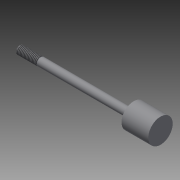
# Autodesk Inventor part: 021-DXP0000_rod
Saved by Autodesk Inventor 2014 SP2 (Build 180246200, 246)
## iProperties
Created: 2019-01-18
Part Number: 021-DXP0000_rod
Material: Generic
Catalog Web Link: www.cadenas.de
Description: Standard Air Cylinder_rod-Original Line - Standard Air Cylinders
Vendor: BIMBA
Document SubType Name: Modeling
Designer: psadmin
Manufacturer: BIMBA
Mass: 3.79157 g
Surface Area: 20.575 cm^2
Volume: 3.79157 cm^3
Density: 1 g/cm^3
Appearance: PSOLRGB-181-181-181
Category: PARTsolutions
Company: BIMBA
Title: 021-DXP0000_rod
Author: Cadenas PARTsolutions
Comments: Original Line - Standard Air Cylinders
PSOL_IDENT_0: {$CADENAS_DATA\23d-libs\bimba\bimba\bimba_imperial\bimba_full_line\original_line_cylinders\standard_
PSOL_IDENT_1: air_cylinders\rod.prj},323 {VTYP=3D},{NB=021-DXP0000_rod},{LINA=021-DXP0000_rod},{NN=Standard Air Cy
PSOL_IDENT_2: linder_rod},{DATE=21.03.2018 14:31:21},{GEOMDATE=09.11.2017 13:09:15},{VERSION=},{LINEID=40},{WBVAR=
PSOL_IDENT_3: STROKE,ACTING,MNT,DER,NR,BM,CO,M,EE,EEL,K,Q,Y,F,G,T,B,H,SER,SR,NT,W,E,HL,ST,STP,PRC,PB,COLOR1,FCD,RC
PSOL_IDENT_4: D,BCD},{WBNUMERIC=STROKE,EEL,COLOR1,FCD,RCD,BCD}  {NB=021-DXP0000_rod},{LINA=021-DXP0000_rod},{KT=DU
PSOL_IDENT_5: MMY},{PN=021-DXP000},{DASH=-},{BORE=0.56250000},{BOREPN=02},{STROKE=1.000},{STROKEALG=[0.001:50/0.00
PSOL_IDENT_6: 1]},{STROKE1=1.000},{ACTING=D},{ACTINGALG= '' , 'Single Acting' , 'R' , 'Reverse Single Acting' , 'D'
PSOL_IDENT_7: , 'Double Acting' },{ACTINGPN=D},{MNT=XP},{MNTALG= '' , 'Front Nose Mounting' , 'XP' , 'Double End
PSOL_IDENT_8: or Rear Pivot Mounting' , 'X' , 'Double End Mounting' },{TYPE=},{MNTPN=XP},{DER=},{DERALG= '' , 'N/A'
PSOL_IDENT_9: },{NR=},{NRALG= '' , 'N/A' },{NRPN=},{BM=},{BMALG= '' , 'N/A' },{BMPN=},{CO=},{COALG= '' , 'N/A' },
PSOL_IDENT_10: {M=},{MALG= '', 'Without Magnet', 'M', 'With Magnet' },{EE=},{EEL=0},{EEMAX=49},{EEALG= '', 'Without
PSOL_IDENT_11: Extra Extension', 'EE', 'With Extra Extension' },{EELALG=0},{EEPN=},{EEPN1=0.000},{K=},{KALG= '', '
PSOL_IDENT_12: Standard' , 'K' , 'Ports Rotated 90deg' },{KPN=},{Q=},{QALG= '' , 'Without Side Ported Rear Head' , '
PSOL_IDENT_13: Q' , 'With Side Ported Rear Head' },{QPN=},{Y=},{YALG= '' , 'With Pivot Bushing' },{YPN=},{F=},{FALG=
PSOL_IDENT_14: '', 'Standard', 'F', 'Molycoated Body' },{FPN=},{G=},{GPN=},{T=},{TALG= '' , 'Standard' , 'N' , 'Lo
PSOL_IDENT_15: w Temperature' , 'V' , 'High Temperature' },{NPN=},{VPN=},{B=},{BALG= '', 'Without Bumper' , 'B' , '
PSOL_IDENT_16: With Bumper' },{BPN=},{H=},{HALG= '', 'N/A' },{HPN=},{SER=},{SERALG= '' , 'Without Spring Extend/Ret
PSOL_IDENT_17: urn' , 'JS' , 'With Spring Return' , 'JR' , 'With Spring Extend' },{SR=},{SRALG= 'C' , 'Carbon Steel
PSOL_IDENT_18: Rod' , 'SR' , '303 Stainless Steel Rod' , '' , '303 Stainless Steel Rod1' },{SRPN=},{SRCON=0},{NT=}
PSOL_IDENT_19: ,{NTPN=},{W=},{WALG= '' , 'Without Wiper' , 'W' , 'With Wiper' },{WPN=},{E=},{EALG= '' , 'Without Sp
PSOL_IDENT_20: ecial Lube and Seals' , 'E' , 'With Special Lube and Seals' },{EPN=},{HL=},{HLALG= '' , 'Wihout Low
PSOL_IDENT_21: Pressure Hydraulic' , 'HL' , 'With Low Pressure Hydraulic' },{ST=},{STALG= '' , 'Without Switch Trac
PSOL_IDENT_22: k' , 'T' , 'With Switch Track' },{STP=},{STPALG= '' , 'N/A' },{STPN=},{PRC=},{PRCALG= '' , 'Without
PSOL_IDENT_23: Piston Rod Clevis' , 'D-166-1' , 'With Piston Rod Clevis' },{PRCPN=},{PB=},{PBALG= '' , 'Without Piv
PSOL_IDENT_24: ot Bracket' , 'D-167' , 'With Pivot Bracket' },{PBPN=},{TLEN=1.8870},{TEXT=0.166667},{SPACE=0.095238
PSOL_IDENT_25: },{FRAC=3.5600},{RGCON=},{RGDACCON=R},{RHCON=P},{RHCONON=1},{RHACCON=R},{FNUTCON=1},{RNUTCON=1},{FNU
PSOL_IDENT_26: TPN=D-154},{RNUTPN=},{FNUTTRANS=0.0000},{RNUTTRANS=0.0000},{VHOLECON=0},{A1=1.1560},{A1N=1.0310},{A1
PSOL_IDENT_27: P=1.1560},{A1B=0.0000},{A4=0.1570},{A4N=0.5310},{A4P=0.1570},{A5=0.0250},{A1H=0.969},{A1NH=0.5000},{
PSOL_IDENT_28: A1PH=0.9690},{A1BH=0.0000},{A1SH=0.0000},{A2H=0.1570},{A2NH=0.1570},{LENGTH=2.5600},{LENGTH1=2.5600}
PSOL_IDENT_29: ,{LENGTH2=2.6100},{MUL=1.0000},{MUL11=1.0000},{MUL22=2.6300},{MUL33=1.6300},{MUL2=1.0000},{MUL211=1.
PSOL_IDENT_30: 0000},{MUL222=2.6300},{MUL233=1.6300},{SSS=2.0000},{RGLEN=1.0240},{RHLEN=0.6490},{SSS1=2.0000},{A13=
PSOL_IDENT_31: 0.7810},{THDLEN1=0.5000},{THD1=0.1900},{TAB=UNF},{THDLEN=0.5000},{THD=0.1900},{OD=0.5725},{RODL=3.27
PSOL_IDENT_32: 90},{PL=0.6230},{RODDIA=0.1870},{HEX=0.1870},{RODTRANS=0.0000},{G1=0.0000},{ON=0},{G5=0.0000},{DERLE
PSOL_IDENT_33: N=2.6560},{THOLE=0.0000},{WF=0.0000},{BADD=0.0000},{MADD=0.0000},{NVADD=0.000},{JRADD=0.00000},{COLO
PSOL_IDENT_34: R=0.71,0.71,0.71,0.00},{GROOVE=1},{HOL=0},{D7=0.1570},{H1=0.0000},{D1=0.6150},{D1RH=0.6150},{D1P=0.0
PSOL_IDENT_35: 000},{D1B=0.6150},{D1N=0.6150},{D1NRH=0.6095},{D1BRH=0.0000},{D1PRH=0.6150},{BOZO=0},{HADD=0.000},{C
PSOL_IDENT_36: OLOR1=0},{DEFL=0.0000},{HEXL=0.0000},{SSADD=0.0000},{WFL=0.0000},{MOVE=0.0000},{PRCL2=0.37500},{PRCB=
PSOL_IDENT_37: 0.12000},{PRCTRANS=0.00000},{FCD=0},{RCD=0},{BCD=0}
NN: Standard Air Cylinder_rod
NT: Standard
NB: 021-DXP0000_rod
NBSYN: $PN.$COLOR1._rod
LINA: 021-DXP0000_rod
PN: 021-DXP000
BORE: 0.5625
BOREPN: 02
STROKE: 1
ACTING: Double Acting
MNT: Double End or Rear Pivot Mounting
DER: N/A
NR: N/A
BM: N/A
CO: N/A
M: Without Magnet
EE: Without Extra Extension
EEL: 0
K: Standard
Q: Without Side Ported Rear Head
Y: With Pivot Bushing
F: Standard
G: Without Magnalube Lubrication
T: Standard
B: Without Bumper
H: N/A
SER: Without Spring Extend/Return
SR: 303 Stainless Steel Rod1
W: Without Wiper
E: Without Special Lube and Seals
HL: Wihout Low Pressure Hydraulic
ST: Without Switch Track
STP: N/A
PRC: Without Piston Rod Clevis
PB: Without Pivot Bracket
A1N: 1.031
A1P: 1.156
A1B: 0
A4N: 0.531
A4P: 0.157
A5: 0.025
A1NH: 0.5
A1PH: 0.969
A1BH: 0
A1SH: 0
A2NH: 0.157
A13: 0.781
THDLEN1: 0.5
THD1: 0.19
TAB: UNF
OD: 0.5725
RODDIA: 0.187
HEX: 0.187
G1: 0
G5: 0
THOLE: 0
WF: 0
GROOVE: 1
D7: 0.157
D1P: 0
D1B: 0.615
D1N: 0.615
D1NRH: 0.6095
D1BRH: 0
D1PRH: 0.615
COLOR1: 0
FCD: 0
RCD: 0
BCD: 0
SUPPLIER: BIMBA
ARTICLENO: 021-DXP0000_rod
BOMINFO: 021-DXP0000_rod
CREATOR: CADENAS GmbH
Autodesk Inventor part; units mm, degrees
ref_plane "YZ Plane" through (0, 0, 0) normal (1, 0, 0) x (0, 1, 0)
ref_plane "XZ Plane" through (0, 0, 0) normal (0, 1, 0) x (-1, 0, 0)
ref_plane "XY Plane" through (0, 0, 0) normal (0, 0, 1) x (1, 0, 0)
sketch "Sketch_1" plane through (0, 0, 0) normal (0, 0, 1) x (1, 0, 0)
  line L0 (70.5866, 0) -> (0, 0)
  line L1 (0, 0) -> (0, 2.3749)
  line L2 (0, 2.3749) -> (54.7624, 2.3749)
  line L3 (54.7624, 2.3749) -> (54.7624, 7.22)
  line L4 (54.7624, 7.22) -> (70.5866, 7.22)
  line L5 (70.5866, 7.22) -> (70.5866, 0)
  line L6 (70.5866, 0) -> (0, 0)
  constraints: 14 end point
revolve "Revolution1" add sketch "Sketch_1" angle 360 about axis through (70.5866, 0, 0) along (1, 0, 0)
sketch "Sketch_3" plane through (0, 0, 0) normal (0, 0, 1) x (1, 0, 0)
  line L0 (0, 0) -> (-12.7, 0)
  line L1 (-12.7, 0) -> (-12.7, 1.9406)
  line L2 (-12.7, 1.9406) -> (-12.2276, 2.413)
  line L3 (-12.2276, 2.413) -> (0, 2.413)
  line L4 (0, 2.413) -> (0, 0)
  line L5 (0, 0) -> (-12.7, 0)
  constraints: 12 end point
revolve "Revolution2" add sketch "Sketch_3" angle 360 about axis through (0, 0, 0) along (1, 0, 0)
thread "Thread1" size "10-32 UNF" class "2A" standard "ANSI Unified Screw Threads" full length
sketch "Sketch_30" plane through (0, 0, 0) normal (0, 0, 1) x (1, 0, 0)
  line L0 (0, 0) -> (-0.254, 0)
  line L1 (-0.254, 2.159) -> (0, 2.159)
  line L2 (0, 2.159) -> (0, 2.667)
  line L3 (0, 2.667) -> (-0.254, 2.667)
  line L4 (-0.254, 2.667) -> (-0.254, 2.159)
  constraints: 10 end point
revolve "Revolution3" cut sketch "Sketch_30" angle 360 about axis through (0, 0, 0) along (1, 0, 0)
ref_plane "dia1_XY" through (0, 2.3749, 0) normal (1, 0, 0) x (0, 0, -1)
ref_plane "dia1_YZ" through (0, 2.3749, 0) normal (0, 0, -1) x (0, 1, 0)
ref_plane "dia1_ZX" through (0, 2.3749, 0) normal (0, 1, 0) x (1, 0, 0)
ref_plane "dia12_XY" through (0, 0, 7.8105) normal (1, 0, 0) x (0, 0, -1)
ref_plane "dia12_YZ" through (0, 0, 7.8105) normal (0, 0, -1) x (0, 1, 0)
ref_plane "dia12_ZX" through (0, 0, 7.8105) normal (0, 1, 0) x (1, 0, 0)
ref_plane "dia2_XY" through (0, -2.3749, 0) normal (1, 0, 0) x (0, 0, -1)
ref_plane "dia2_YZ" through (0, -2.3749, 0) normal (0, 0, -1) x (0, 1, 0)
ref_plane "dia2_ZX" through (0, -2.3749, 0) normal (0, 1, 0) x (1, 0, 0)
ref_plane "dia22_XY" through (0, 0, -7.8105) normal (1, 0, 0) x (0, 0, -1)
ref_plane "dia22_YZ" through (0, 0, -7.8105) normal (0, 0, -1) x (0, 1, 0)
ref_plane "dia22_ZX" through (0, 0, -7.8105) normal (0, 1, 0) x (1, 0, 0)
ref_plane "rl1_XY" through (-12.7, 0, 0) normal (1, 0, 0) x (0, 0, -1)
ref_plane "rl1_YZ" through (-12.7, 0, 0) normal (0, 0, -1) x (0, 1, 0)
ref_plane "rl1_ZX" through (-12.7, 0, 0) normal (0, 1, 0) x (1, 0, 0)
ref_plane "rl2_XY" through (0, 0, 0) normal (1, 0, 0) x (0, 0, -1)
ref_plane "rl2_YZ" through (0, 0, 0) normal (0, 0, -1) x (0, 1, 0)
ref_plane "rl2_ZX" through (0, 0, 0) normal (0, 1, 0) x (1, 0, 0)
ref_plane "rod_cp_XY" through (0, 0, 0) normal (1, 0, 0) x (0, 0, -1)
ref_plane "rod_cp_YZ" through (0, 0, 0) normal (0, 0, -1) x (0, 1, 0)
ref_plane "rod_cp_ZX" through (0, 0, 0) normal (0, 1, 0) x (1, 0, 0)
ref_plane "thd1_XY" through (-12.7, 2.413, 0) normal (1, 0, 0) x (0, 0, -1)
ref_plane "thd1_YZ" through (-12.7, 2.413, 0) normal (0, 0, -1) x (0, 1, 0)
ref_plane "thd1_ZX" through (-12.7, 2.413, 0) normal (0, 1, 0) x (1, 0, 0)
ref_plane "thd2_XY" through (-12.7, -2.413, 0) normal (1, 0, 0) x (0, 0, -1)
ref_plane "thd2_YZ" through (-12.7, -2.413, 0) normal (0, 0, -1) x (0, 1, 0)
ref_plane "thd2_ZX" through (-12.7, -2.413, 0) normal (0, 1, 0) x (1, 0, 0)
ref_plane "to_rod_clevis_XY" through (-12.7, 0, 0) normal (1, 0, 0) x (0, 0, -1)
ref_plane "to_rod_clevis_YZ" through (-12.7, 0, 0) normal (0, 0, -1) x (0, 1, 0)
ref_plane "to_rod_clevis_ZX" through (-12.7, 0, 0) normal (0, 1, 0) x (1, 0, 0)
body "Solid1"
